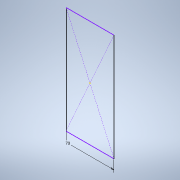
# Autodesk Inventor part: top lid
Saved by Autodesk Inventor 2020 (Build 240168000, 168)
## iProperties
Created: 2022-02-16
Part Number: top lid
Material: Generic
Document SubType Name: Modeling
Designer: rwte
Density: 1 g/cm^3
Appearance: Default
Author: rwte
Autodesk Inventor part; units mm, degrees
ref_plane "YZ Plane" through (0, 0, 0) normal (1, 0, 0) x (0, 1, 0)
ref_plane "XZ Plane" through (0, 0, 0) normal (0, 1, 0) x (-1, 0, 0)
ref_plane "XY Plane" through (0, 0, 0) normal (0, 0, 1) x (1, 0, 0)
sketch "Sketch1" plane through (0, 0, 0) normal (0, 0, 1) x (1, 0, 0)
  line L0 (-37, -40.5) -> (-37, 40.5)
  line L1 (-37, 40.5) -> (37, 40.5)
  line L2 (37, 40.5) -> (37, -40.5)
  line L3 (37, -40.5) -> (-37, -40.5)
  line L4 (-37, -40.5) -> (37, 40.5) construction
  line L5 (-37, 40.5) -> (37, -40.5) construction
  point P0 (0, 0)
  dimension "d0" = 74
  dimension "d1" = 81
  constraints: 12 end point, 2 midpoint, 2 parallel, 1 perpendicular, 1 vertical
  measures "d0" distance of L2.end L0.start
  measures "d1" distance of L1.end L2.end
extrude "Extrusion1" add sketch "Sketch1" along normal blind 3
body "Solid1"
